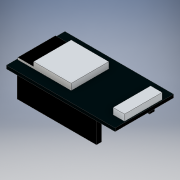
# Autodesk Inventor part: ESP32
Saved by Autodesk Inventor 2019 (Build 230136000, 136)
## iProperties
Created: 2022-02-03
Part Number: ESP32
Material: Generic
Document SubType Name: Modeling
Designer: josec
Density: 1 g/cm^3
Appearance: Default
Author: josec
Autodesk Inventor part; units mm, degrees
ref_plane "YZ Plane" through (0, 0, 0) normal (1, 0, 0) x (0, 1, 0)
ref_plane "XZ Plane" through (0, 0, 0) normal (0, 1, 0) x (-1, 0, 0)
ref_plane "XY Plane" through (0, 0, 0) normal (0, 0, 1) x (1, 0, 0)
sketch "Sketch1" plane through (0, 0, 0) normal (0, 1, 0) x (-1, 0, 0)
  line L0 (0, 0) -> (-52, 0)
  line L1 (-52, 0) -> (-52, -28)
  line L2 (-52, -28) -> (0, -28)
  line L3 (0, -28) -> (0, 0)
  dimension "d0" = 52
  dimension "d1" = 28
  constraints: 8 end point, 2 parallel, 1 horizontal, 1 perpendicular
  measures "d0" distance of L2.end L1.end
  measures "d1" distance of L1.end L0.end
extrude "Extrusion1" add sketch "Sketch1" along normal blind 1.5
sketch "Sketch2" plane through (0, 1.5, 0) normal (0, 1, 0) x (1, 0, 0)
  line L0 (0, 0) -> (0, 5) construction
  line L1 (0, 28) -> (0, 0) construction
  line L2 (0, 28) -> (0, 23) construction
  line L3 (0, 23) -> (8, 23)
  line L4 (8, 23) -> (8, 5)
  line L5 (8, 5) -> (0, 5)
  line L6 (0, 5) -> (0, 23)
  dimension "d4" = 5
  dimension "d5" = 5
  dimension "d6" = 8
  constraints: 12 end point, 2 parallel, 2 point on line, 1 horizontal, 1 perpendicular
  measures "d4" distance of L0.start L0.end
  measures "d5" distance of L1.start L2.end
  measures "d6" distance of L4.end L5.end
extrude "Extrusion2" add sketch "Sketch2" along normal blind 1
sketch "Sketch3" plane through (0, 1.5, 0) normal (0, 1, 0) x (1, 0, 0)
  line L0 (8, 5) -> (8, 23) projected
  line L1 (8, 23) -> (26, 23)
  line L2 (26, 23) -> (26, 5)
  line L3 (26, 5) -> (8, 5)
  line L4 (8, 5) -> (8, 23)
  point P0 (0, 0)
  dimension "d9" = 18
  constraints: 8 end point, 2 parallel, 1 horizontal, 1 perpendicular
  measures "d9" distance of L2.end L3.end
extrude "Extrusion3" add sketch "Sketch3" along normal blind 3
sketch "Sketch4" plane through (0, 1.5, 0) normal (0, 1, 0) x (1, 0, 0)
  line L0 (52, 28) -> (52, 23) construction
  line L1 (52, 0) -> (52, 28) construction
  line L2 (52, 0) -> (52, 5) construction
  line L3 (52, 23) -> (46, 23)
  line L4 (46, 23) -> (46, 5)
  line L5 (46, 5) -> (52, 5)
  line L6 (52, 5) -> (52, 23)
  point P0 (0, 0)
  dimension "d12" = 5
  dimension "d13" = 5
  dimension "d14" = 6
  constraints: 12 end point, 2 parallel, 2 point on line, 1 horizontal, 1 perpendicular
  measures "d12" distance of L0.start L0.end
  measures "d13" distance of L1.start L2.end
  measures "d14" distance of L5.end L4.end
extrude "Extrusion4" add sketch "Sketch4" along normal blind 3
sketch "Sketch5" plane through (52, 0, 0) normal (1, 0, 0) x (0, 0, -1)
  line L0 (5, 4.5) -> (23, 4.5) projected
  line L1 (23, 1.5) -> (28, 1.5) projected
  line L2 (5, 4.5) -> (23, 4.5)
  line L3 (23, 4.5) -> (23, 1.5)
  line L4 (23, 1.5) -> (5, 1.5)
  line L5 (5, 1.5) -> (5, 4.5)
  point P0 (0, 0)
  constraints: 8 end point, 2 parallel, 1 horizontal, 1 perpendicular
extrude "Extrusion5" cut sketch "Sketch5" against normal blind 0.5
sketch "Sketch6" plane through (0, 0, -28) normal (-1, 0, 0) x (0, 0, 1)
  line L0 (5, 2.5) -> (23, 2.5) projected
  line L1 (23, 1.5) -> (5, 1.5) projected
  line L2 (5, 2.5) -> (23, 2.5)
  line L3 (23, 2.5) -> (23, 1.5)
  line L4 (23, 1.5) -> (5, 1.5)
  line L5 (5, 1.5) -> (5, 2.5)
  point P0 (28, 0)
  constraints: 8 end point, 2 parallel, 1 horizontal, 1 perpendicular
extrude "Extrusion6" cut sketch "Sketch6" against normal blind 0.5
sketch "Sketch7" plane through (0, 0, 0) normal (0, -1, 0) x (1, 0, 0)
  line L0 (0, -28) -> (0, 0) construction
  line L1 (0, 0) -> (5, 0) construction
  line L2 (0, 0) -> (52, 0) construction
  line L3 (52, 0) -> (43, 0) construction
  line L4 (5, 0) -> (43, 0)
  line L5 (43, 0) -> (43, -2.5)
  line L6 (43, -2.5) -> (5, -2.5)
  line L7 (5, -2.5) -> (5, 0)
  line L8 (52, -28) -> (0, -28) projected
  line L9 (5, -28) -> (43, -28)
  line L10 (43, -28) -> (43, -25.5)
  line L11 (43, -25.5) -> (5, -25.5)
  line L12 (5, -25.5) -> (5, -28)
  dimension "d21" = 5
  dimension "d22" = 9
  dimension "d23" = 2.5
  dimension "d24" = 2.5
  constraints: 20 end point, 4 parallel, 3 point on line, 2 horizontal, 2 perpendicular
  measures "d21" distance of L0.end L1.end
  measures "d22" distance of L2.end L3.end
  measures "d23" distance of L4.end L5.end
  measures "d24" distance of L10.end L9.end
extrude "Extrusion7" add sketch "Sketch7" along normal blind 10
sketch "Sketch8" plane through (52, 1.5, -28) normal (0, 0, -1) x (-1, 0, 0)
  line L0 (47, -11.5) -> (9, -11.5) projected
  line L1 (9, -1.5) -> (9, -11.5) projected
  line L2 (47, -11.5) -> (9, -11.5)
  line L3 (9, -11.5) -> (9, -1.5)
  line L4 (9, -1.5) -> (47, -1.5)
  line L5 (47, -1.5) -> (47, -11.5)
  point P0 (52, -1.5)
  constraints: 8 end point, 2 parallel, 1 horizontal, 1 perpendicular
extrude "Extrusion8" cut sketch "Sketch8" against normal blind 0.1
sketch "Sketch9" plane through (0, 1.5, 0) normal (0, 0, 1) x (1, 0, 0)
  line L0 (5, -1.5) -> (5, -11.5) projected
  line L1 (43, -11.5) -> (43, -1.5) projected
  line L2 (5, -1.5) -> (43, -1.5)
  line L3 (43, -1.5) -> (43, -11.5)
  line L4 (43, -11.5) -> (5, -11.5)
  line L5 (5, -11.5) -> (5, -1.5)
  point P0 (0, -1.5)
  constraints: 8 end point, 2 parallel, 1 horizontal, 1 perpendicular
extrude "Extrusion9" cut sketch "Sketch9" against normal blind 0.1
body "Solid1"
